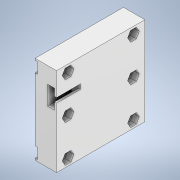
# Autodesk Inventor part: XItemEndCoverConnector
Saved by Autodesk Inventor 2020 (Build 240168000, 168)
## iProperties
Created: 2022-03-12
Part Number: XItemEndCoverConnector
Material: Tworzywo sztuczne ABS
Document SubType Name: Modeling
Designer: mikoma
Density: 1.06 g/cm^3
Appearance: Gładki — biały
Mass: 52.637 g
Surface Area: 154.031 cm^2
Volume: 49.6575 cm^3
Author: mikoma
Autodesk Inventor part; units mm, degrees
ref_plane "YZ Plane" through (0, 0, 0) normal (1, 0, 0) x (0, 1, 0)
ref_plane "XZ Plane" through (0, 0, 0) normal (0, 1, 0) x (-1, 0, 0)
ref_plane "XY Plane" through (0, 0, 0) normal (0, 0, 1) x (1, 0, 0)
sketch "Szkic1" plane through (0, 0, 0) normal (1, 0, 0) x (0, 1, 0)
  line L0 (-37, 37) -> (37, 37)
  line L1 (37, 37) -> (37, -37)
  line L2 (37, -37) -> (-37, -37)
  line L3 (-37, -37) -> (-37, 37)
  line L4 (-37, 37) -> (37, -37) construction
  line L5 (37, 37) -> (-37, -37) construction
  point P0 (0, 0)
  dimension "d0" = 74
  dimension "d1" = 74
  constraints: 12 end point, 2 midpoint, 2 parallel, 1 horizontal, 1 perpendicular
  measures "d0" distance of L0.end L1.end
  measures "d1" distance of L1.end L2.end
extrude "Wyciągnięcie proste1" add sketch "Szkic1" along normal blind 18
sketch "Szkic2" plane through (18, 0, 0) normal (1, 0, 0) x (0, 0, -1)
  circle A0 centre (-27.4, 31) radius 2.85
  line L0 (37, 37) -> (-37, 37) projected
  line L1 (-37, 37) -> (-37, -37) projected
  circle A1 centre (-27.4, 0) radius 2.85
  circle A2 centre (-27.4, -31) radius 2.85
  circle A3 centre (27.4, 31) radius 2.85
  line L2 (37, -37) -> (37, 37) projected
  circle A4 centre (27.4, 0) radius 2.85
  circle A5 centre (27.4, -31) radius 2.85
  line L3 (-29.8537, 35.25) -> (-24.9463, 35.25)
  line L4 (-24.9463, 35.25) -> (-22.4925, 31)
  line L5 (-22.4925, 31) -> (-24.9463, 26.75)
  line L6 (-24.9463, 26.75) -> (-29.8537, 26.75)
  line L7 (-29.8537, 26.75) -> (-32.3075, 31)
  line L8 (-32.3075, 31) -> (-29.8537, 35.25)
  line L9 (-29.8537, 4.25) -> (-24.9463, 4.25)
  line L10 (-24.9463, 4.25) -> (-22.4925, 0)
  line L11 (-22.4925, 0) -> (-24.9463, -4.25)
  line L12 (-24.9463, -4.25) -> (-29.8537, -4.25)
  line L13 (-29.8537, -4.25) -> (-32.3075, 0)
  line L14 (-32.3075, 0) -> (-29.8537, 4.25)
  line L15 (-29.8537, -26.75) -> (-24.9463, -26.75)
  line L16 (-24.9463, -26.75) -> (-22.4925, -31)
  line L17 (-22.4925, -31) -> (-24.9463, -35.25)
  line L18 (-24.9463, -35.25) -> (-29.8537, -35.25)
  line L19 (-29.8537, -35.25) -> (-32.3075, -31)
  line L20 (-32.3075, -31) -> (-29.8537, -26.75)
  line L21 (29.8537, 35.25) -> (32.3075, 31)
  line L22 (32.3075, 31) -> (29.8537, 26.75)
  line L23 (29.8537, 26.75) -> (24.9463, 26.75)
  line L24 (24.9463, 26.75) -> (22.4925, 31)
  line L25 (22.4925, 31) -> (24.9463, 35.25)
  line L26 (24.9463, 35.25) -> (29.8537, 35.25)
  line L27 (29.8537, 4.25) -> (32.3075, 0)
  line L28 (32.3075, 0) -> (29.8537, -4.25)
  line L29 (29.8537, -4.25) -> (24.9463, -4.25)
  line L30 (24.9463, -4.25) -> (22.4925, 0)
  line L31 (22.4925, 0) -> (24.9463, 4.25)
  line L32 (24.9463, 4.25) -> (29.8537, 4.25)
  line L33 (29.8537, -26.75) -> (32.3075, -31)
  line L34 (32.3075, -31) -> (29.8537, -35.25)
  line L35 (29.8537, -35.25) -> (24.9463, -35.25)
  line L36 (24.9463, -35.25) -> (22.4925, -31)
  line L37 (22.4925, -31) -> (24.9463, -26.75)
  line L38 (24.9463, -26.75) -> (29.8537, -26.75)
  point P0 (0, 0)
  point P1 (27.4, -26.75)
  dimension "d4" = 6
  dimension "d5" = 5.7
  dimension "d6" = 9.6
  dimension "d7" = 31
  dimension "d8" = 31
  dimension "d9" = 5.7
  dimension "d10" = 5.7
  dimension "d11" = 9.6
  dimension "d12" = 5.7
  dimension "d13" = 5.7
  dimension "d14" = 5.7
  dimension "d15" = 8.5
  dimension "d16" = 8.5
  dimension "d17" = 8.5
  dimension "d18" = 8.5
  dimension "d19" = 8.5
  dimension "d20" = 8.5
  constraints: 72 end point, 6 centre point, 6 coincident, 6 horizontal, 4 vertical alignment, 3 horizontal alignment, 1 midpoint, 78 other
  measures "d4" distance from line of L0 A0.centre
  measures "d5" diameter of A0
  measures "d6" distance from line of L1 A0.centre
  measures "d7" distance of A0.centre A1.centre
  measures "d8" distance of A2.centre A1.centre
  measures "d9" diameter of A1
  measures "d10" diameter of A2
  measures "d11" distance from line of L2 A3.centre
  measures "d12" diameter of A3
  measures "d13" diameter of A4
  measures "d14" diameter of A5
  measures "d15" distance of L6.end L3.start
  measures "d16" distance of L9.start L12.end
  measures "d17" distance between parallel lines of L18 L15
  measures "d18" distance between parallel lines of L23 L26
  measures "d19" distance between parallel lines of L29 L32
  measures "d20" distance between parallel lines of L35 L38
extrude "Wyciągnięcie proste2" cut sketch "Szkic2" against normal through all contours A0 | A1 | A2 | A3 | A4 | A5
extrude "Wyciągnięcie proste3" cut sketch "Szkic2" against normal blind 5 contours A0 | A1 | A2 | A3 | A4 | A5 | L3 L4 L5 L6 L7 L8 | L9 L10 L11 L12 L13 L14 | L15 L16 L17 L18 L19 L20 | L21 L22 L23 L24 L25 L26 | L27 L28 L29 L30 L31 L32 | L33 L34 L35 L36 L37 L38
sketch "Szkic3" plane through (0, -37, 37) normal (0, 0, 1) x (1, 0, 0)
  line L0 (0, 0) -> (0, 74) projected
  line L1 (0, 72.5) -> (2, 72.5)
  line L2 (2, 72.5) -> (2, 63.5)
  line L3 (2, 63.5) -> (0, 63.5)
  line L4 (0, 63.5) -> (0, 72.5)
  line L5 (0, 74) -> (18, 74) projected
  line L6 (0, 10.5) -> (2, 10.5)
  line L7 (2, 10.5) -> (2, 1.5)
  line L8 (2, 1.5) -> (0, 1.5)
  line L9 (0, 1.5) -> (0, 10.5)
  point P0 (0, 37)
  point P1 (0, 1.5)
  point P2 (0, 63.5)
  dimension "d25" = 1.5
  dimension "d26" = 9
  dimension "d27" = 2
  dimension "d28" = 2
  dimension "d29" = 9
  dimension "d30" = 1.5
  constraints: 16 end point, 4 parallel, 2 horizontal, 2 perpendicular, 2 point on line
  measures "d25" distance between parallel lines of L1 L5
  measures "d26" distance of L1.end L2.end
  measures "d27" distance between parallel lines of L0 L2
  measures "d28" distance of L6.start L6.end
  measures "d29" distance of L6.end L7.end
  measures "d30" distance from line of L8 L0.start
extrude "Wyciągnięcie proste4" cut sketch "Szkic3" against normal through all
sketch "Szkic4" plane through (0, -37, 37) normal (0, 0, 1) x (1, 0, 0)
  line L0 (10.5, 60.5) -> (10.5, 44.5)
  line L1 (10.5, 44.5) -> (16.3, 44.5)
  line L2 (16.3, 44.5) -> (16.3, 50.5)
  line L3 (16.3, 60.5) -> (10.5, 60.5)
  line L4 (16.3, 50.5) -> (18, 50.5)
  line L5 (18, 50.5) -> (18, 54.5)
  line L6 (18, 54.5) -> (16.3, 54.5)
  line L7 (16.3, 54.5) -> (16.3, 60.5)
  line L8 (16.3, 50.5) -> (16.3, 54.5) construction
  line L9 (18, 74) -> (18, 0) projected
  line L10 (18, 63.75) -> (13, 63.75) projected
  line L11 (18, 63.75) -> (13, 63.75) projected
  point P0 (0, 37)
  dimension "d33" = 5.8
  dimension "d34" = 4
  dimension "d35" = 1.7
  dimension "d36" = 6
  dimension "d37" = 16
  dimension "d38" = 3.25
  constraints: 18 end point, 6 parallel, 1 horizontal, 1 perpendicular, 1 point on line
  measures "d33" distance of L0.end L1.end
  measures "d34" distance of L4.end L5.end
  measures "d35" distance of L2.end L4.end
  measures "d36" distance between parallel lines of L1 L4
  measures "d37" distance of L0.start L0.end
  measures "d38" distance between parallel lines of L3 L11
extrude "Wyciągnięcie proste5" cut sketch "Szkic4" against normal blind 20
